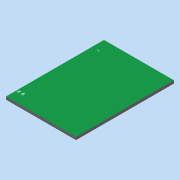
# Autodesk Inventor part: mezzaninePCB
Saved by Autodesk Inventor 2016 (Build 200138000, 138)
## iProperties
Created: 2016-08-31
Part Number: mezzaninePCB
Material: Generic
Document SubType Name: Modeling
Designer: Zara
Density: 1 g/cm^3
Appearance: Default
Author: Zara
Autodesk Inventor part; units mm, degrees
ref_plane "YZ Plane" through (0, 0, 0) normal (1, 0, 0) x (0, 1, 0)
ref_plane "XZ Plane" through (0, 0, 0) normal (0, 1, 0) x (-1, 0, 0)
ref_plane "XY Plane" through (0, 0, 0) normal (0, 0, 1) x (1, 0, 0)
sketch "Sketch1" plane through (0, 0, 0) normal (0, 1, 0) x (-1, 0, 0)
  line L0 (-25, 35) -> (25, 35)
  line L1 (25, 35) -> (25, -35)
  line L2 (25, -35) -> (-25, -35)
  line L3 (-25, -35) -> (-25, 35)
  line L4 (-25, 35) -> (25, -35) construction
  line L5 (25, 35) -> (-25, -35) construction
  point P0 (0, 0)
  dimension "d0" = 70
  dimension "d1" = 50
  constraints: 12 end point, 2 midpoint, 2 parallel, 1 horizontal, 1 perpendicular
  measures "d0" distance of L0.end L1.end
  measures "d1" distance of L1.end L2.end
extrude "Extrusion1" add sketch "Sketch1" along normal blind 2
sketch "Sketch2" plane through (0, 2, 0) normal (0, 1, 0) x (1, 0, 0)
  line L0 (-19.9573, 27.2181) -> (-19.9573, 24.5917) construction
  line L1 (-19.9573, 24.5917) -> (-23.5311, 24.5917) construction
  line L2 (-23.5311, 24.5917) -> (-23.5311, 27.2181) construction
  line L3 (-23.5311, 27.2181) -> (-19.9573, 27.2181) construction
  line L4 (-23.2113, -25.6951) -> (-23.2113, -28.3215) construction
  line L5 (-23.2113, -28.3215) -> (-19.3854, -28.3215) construction
  line L6 (-19.3854, -28.3215) -> (-19.3854, -25.6951) construction
  line L7 (-19.3854, -25.6951) -> (-23.2113, -25.6951) construction
  line L8 (-19.9654, -25.6528) -> (-19.9654, -28.2792) construction
  line L9 (-19.9654, -28.2792) -> (-23.5391, -28.2792) construction
  line L10 (-23.5391, -28.2792) -> (-23.5391, -25.6528) construction
  line L11 (-23.5391, -25.6528) -> (-19.9654, -25.6528) construction
  line L12 (-21.489, 26.1837) -> (-21.489, 27.1087)
  line L13 (-21.489, 27.1087) -> (-21.2762, 27.1087)
  spline S0 degree 2 poles (-21.2762, 27.1087) (-21.1826, 27.0091) (-21.0088, 26.8316) (-20.9152, 26.7465) knots 0 0 0 1 2 2 2
  spline S1 degree 2 poles (-20.9152, 26.7465) (-20.7268, 26.5751) (-20.5007, 26.4499) (-20.3804, 26.4499) knots 0 0 0 1 2 2 2
  spline S2 degree 2 poles (-20.3804, 26.4499) (-20.3172, 26.4499) (-20.2223, 26.4888) (-20.1919, 26.5241) knots 0 0 0 1 2 2 2
  spline S3 degree 2 poles (-20.1919, 26.5241) (-20.1616, 26.5593) (-20.1312, 26.6517) (-20.1312, 26.7076) knots 0 0 0 1 2 2 2
  spline S4 degree 2 poles (-20.1312, 26.7076) (-20.1312, 26.7611) (-20.1579, 26.8705) (-20.1786, 26.9203) knots 0 0 0 1 2 2 2
  spline S5 degree 2 poles (-20.1786, 26.9203) (-20.1956, 26.9629) (-20.2442, 27.0419) (-20.2612, 27.0662) knots 0 0 0 1 2 2 2
  line L14 (-20.2612, 27.0662) -> (-20.2612, 27.0771)
  line L15 (-20.2612, 27.0771) -> (-20.0473, 27.0771)
  spline S6 degree 2 poles (-20.0473, 27.0771) (-20.0169, 27.0151) (-19.9573, 26.7927) (-19.9573, 26.693) knots 0 0 0 1 2 2 2
  spline S7 degree 2 poles (-19.9573, 26.693) (-19.9573, 26.4827) (-20.1798, 26.2457) (-20.3694, 26.2457) knots 0 0 0 1 2 2 2
  spline S8 degree 2 poles (-20.3694, 26.2457) (-20.4582, 26.2457) (-20.6065, 26.287) (-20.6697, 26.3235) knots 0 0 0 1 2 2 2
  spline S9 degree 2 poles (-20.6697, 26.3235) (-20.7353, 26.36) (-20.8642, 26.4657) (-20.9261, 26.5241) knots 0 0 0 1 2 2 2
  spline S10 degree 2 poles (-20.9261, 26.5241) (-21.0295, 26.6189) (-21.2507, 26.851) (-21.3151, 26.9203) knots 0 0 0 1 2 2 2
  line L16 (-21.3151, 26.9203) -> (-21.3151, 26.1837)
  line L17 (-21.3151, 26.1837) -> (-21.489, 26.1837)
  line L18 (-20.9804, -26.7273) -> (-20.9804, -26.5486)
  line L19 (-20.9804, -26.5486) -> (-21.4958, -26.5486)
  line L20 (-21.4958, -26.5486) -> (-21.4958, -26.3554)
  line L21 (-21.4958, -26.3554) -> (-20.9804, -26.3554)
  line L22 (-20.9804, -26.3554) -> (-20.9804, -25.6929)
  line L23 (-20.9804, -25.6929) -> (-20.7689, -25.6929)
  line L24 (-20.7689, -25.6929) -> (-19.9958, -26.3639)
  line L25 (-19.9958, -26.3639) -> (-19.9958, -26.5486)
  line L26 (-19.9958, -26.5486) -> (-20.8187, -26.5486)
  line L27 (-20.8187, -26.5486) -> (-20.8187, -26.7273)
  line L28 (-20.8187, -26.7273) -> (-20.9804, -26.7273)
  line L29 (-20.8187, -26.3554) -> (-20.2328, -26.3554)
  line L30 (-20.2328, -26.3554) -> (-20.8187, -25.8509)
  line L31 (-20.8187, -25.8509) -> (-20.8187, -26.3554)
  spline S11 degree 2 poles (-20.7458, -27.8213) (-21.1493, -27.8213) (-21.5274, -27.5867) (-21.5274, -27.3424) knots 0 0 0 1 2 2 2
  spline S12 degree 2 poles (-21.5274, -27.3424) (-21.5274, -27.0944) (-21.142, -26.8622) (-20.747, -26.8622) knots 0 0 0 1 2 2 2
  spline S13 degree 2 poles (-20.747, -26.8622) (-20.341, -26.8622) (-19.9654, -27.0969) (-19.9654, -27.3424) knots 0 0 0 1 2 2 2
  spline S14 degree 2 poles (-19.9654, -27.3424) (-19.9654, -27.5892) (-20.3544, -27.8213) (-20.7458, -27.8213) knots 0 0 0 1 2 2 2
  spline S15 degree 2 poles (-21.2028, -27.5636) (-21.1287, -27.5928) (-20.9002, -27.6171) (-20.7458, -27.6171) knots 0 0 0 1 2 2 2
  spline S16 degree 2 poles (-20.7458, -27.6171) (-20.5914, -27.6171) (-20.3641, -27.5928) (-20.2875, -27.5624) knots 0 0 0 1 2 2 2
  spline S17 degree 2 poles (-20.2875, -27.5624) (-20.2109, -27.532) (-20.1319, -27.4263) (-20.1319, -27.3424) knots 0 0 0 1 2 2 2
  spline S18 degree 2 poles (-20.1319, -27.3424) (-20.1319, -27.2585) (-20.2109, -27.1503) (-20.2899, -27.1187) knots 0 0 0 1 2 2 2
  spline S19 degree 2 poles (-20.2899, -27.1187) (-20.3665, -27.0883) (-20.5999, -27.0665) (-20.747, -27.0665) knots 0 0 0 1 2 2 2
  spline S20 degree 2 poles (-20.747, -27.0665) (-20.905, -27.0665) (-21.1165, -27.0859) (-21.1992, -27.1175) knots 0 0 0 1 2 2 2
  spline S21 degree 2 poles (-21.1992, -27.1175) (-21.277, -27.1467) (-21.3608, -27.2549) (-21.3608, -27.3424) knots 0 0 0 1 2 2 2
  spline S22 degree 2 poles (-21.3608, -27.3424) (-21.3608, -27.4251) (-21.2818, -27.5332) (-21.2028, -27.5636) knots 0 0 0 1 2 2 2
  spline S23 degree 2 poles (-23.3852, -26.2093) (-23.3852, -26.1546) (-23.4119, -26.0464) (-23.4326, -25.9941) knots 0 0 0 1 2 2 2
  spline S24 degree 2 poles (-23.4326, -25.9941) (-23.4532, -25.9455) (-23.497, -25.8738) (-23.5165, -25.8458) knots 0 0 0 1 2 2 2
  line L32 (-23.5165, -25.8458) -> (-23.5165, -25.8337)
  line L33 (-23.5165, -25.8337) -> (-23.3037, -25.8337)
  spline S25 degree 2 poles (-23.3037, -25.8337) (-23.2685, -25.8993) (-23.2113, -26.1242) (-23.2113, -26.2251) knots 0 0 0 1 2 2 2
  spline S26 degree 2 poles (-23.2113, -26.2251) (-23.2113, -26.3272) (-23.2527, -26.4791) (-23.2964, -26.5411) knots 0 0 0 1 2 2 2
  spline S27 degree 2 poles (-23.2964, -26.5411) (-23.3438, -26.6067) (-23.4812, -26.6748) (-23.5736, -26.6748) knots 0 0 0 1 2 2 2
  spline S28 degree 2 poles (-23.5736, -26.6748) (-23.6976, -26.6748) (-23.8848, -26.5119) (-23.9091, -26.3977) knots 0 0 0 1 2 2 2
  line L34 (-23.9091, -26.3977) -> (-23.9237, -26.3977)
  spline S29 degree 2 poles (-23.9237, -26.3977) (-23.9334, -26.4451) (-23.9771, -26.5533) (-24.0209, -26.5995) knots 0 0 0 1 2 2 2
  spline S30 degree 2 poles (-24.0209, -26.5995) (-24.0635, -26.6456) (-24.1996, -26.704) (-24.2981, -26.704) knots 0 0 0 1 2 2 2
  spline S31 degree 2 poles (-24.2981, -26.704) (-24.3989, -26.704) (-24.5703, -26.6347) (-24.636, -26.5715) knots 0 0 0 1 2 2 2
  spline S32 degree 2 poles (-24.636, -26.5715) (-24.7041, -26.5059) (-24.7746, -26.3199) (-24.7746, -26.202) knots 0 0 0 1 2 2 2
  spline S33 degree 2 poles (-24.7746, -26.202) (-24.7746, -26.0889) (-24.7199, -25.8677) (-24.6822, -25.7923) knots 0 0 0 1 2 2 2
  line L35 (-24.6822, -25.7923) -> (-24.4694, -25.7923)
  line L36 (-24.4694, -25.7923) -> (-24.4694, -25.8069)
  spline S34 degree 2 poles (-24.4694, -25.8069) (-24.5156, -25.8701) (-24.6007, -26.0841) (-24.6007, -26.1898) knots 0 0 0 1 2 2 2
  spline S35 degree 2 poles (-24.6007, -26.1898) (-24.6007, -26.2518) (-24.5618, -26.3758) (-24.5169, -26.4171) knots 0 0 0 1 2 2 2
  spline S36 degree 2 poles (-24.5169, -26.4171) (-24.4719, -26.4572) (-24.3649, -26.4998) (-24.2835, -26.4998) knots 0 0 0 1 2 2 2
  spline S37 degree 2 poles (-24.2835, -26.4998) (-24.202, -26.4998) (-24.0963, -26.4524) (-24.0659, -26.4098) knots 0 0 0 1 2 2 2
  spline S38 degree 2 poles (-24.0659, -26.4098) (-24.0355, -26.3673) (-24.0124, -26.2518) (-24.0124, -26.1837) knots 0 0 0 1 2 2 2
  line L37 (-24.0124, -26.1837) -> (-24.0124, -26.0986)
  line L38 (-24.0124, -26.0986) -> (-23.8459, -26.0986)
  line L39 (-23.8459, -26.0986) -> (-23.8459, -26.1655)
  spline S39 degree 2 poles (-23.8459, -26.1655) (-23.8459, -26.3004) (-23.717, -26.4706) (-23.5942, -26.4706) knots 0 0 0 1 2 2 2
  spline S40 degree 2 poles (-23.5942, -26.4706) (-23.5371, -26.4706) (-23.4557, -26.4268) (-23.4314, -26.3916) knots 0 0 0 1 2 2 2
  spline S41 degree 2 poles (-23.4314, -26.3916) (-23.4058, -26.3539) (-23.3852, -26.2615) (-23.3852, -26.2093) knots 0 0 0 1 2 2 2
  spline S42 degree 2 poles (-23.7304, -26.8888) (-23.6149, -26.8888) (-23.4229, -26.9641) (-23.3536, -27.0298) knots 0 0 0 1 2 2 2
  spline S43 degree 2 poles (-23.3536, -27.0298) (-23.2867, -27.0918) (-23.2126, -27.2729) (-23.2126, -27.3653) knots 0 0 0 1 2 2 2
  spline S44 degree 2 poles (-23.2126, -27.3653) (-23.2126, -27.4686) (-23.2818, -27.6363) (-23.3475, -27.6983) knots 0 0 0 1 2 2 2
  spline S45 degree 2 poles (-23.3475, -27.6983) (-23.4301, -27.7761) (-23.6976, -27.8612) (-23.903, -27.8612) knots 0 0 0 1 2 2 2
  spline S46 degree 2 poles (-23.903, -27.8612) (-24.089, -27.8612) (-24.422, -27.7773) (-24.5327, -27.6959) knots 0 0 0 1 2 2 2
  spline S47 degree 2 poles (-24.5327, -27.6959) (-24.6494, -27.6096) (-24.7721, -27.3665) (-24.7721, -27.189) knots 0 0 0 1 2 2 2
  spline S48 degree 2 poles (-24.7721, -27.189) (-24.7721, -27.1489) (-24.7636, -27.0577) (-24.7515, -27.0188) knots 0 0 0 1 2 2 2
  line L40 (-24.7515, -27.0188) -> (-24.5582, -27.0188)
  line L41 (-24.5582, -27.0188) -> (-24.5582, -27.0285)
  spline S49 degree 2 poles (-24.5582, -27.0285) (-24.5728, -27.0541) (-24.5983, -27.161) (-24.5983, -27.2157) knots 0 0 0 1 2 2 2
  spline S50 degree 2 poles (-24.5983, -27.2157) (-24.5983, -27.4127) (-24.3382, -27.6375) (-24.0975, -27.6533) knots 0 0 0 1 2 2 2
  spline S51 degree 2 poles (-24.0975, -27.6533) (-24.1522, -27.5731) (-24.202, -27.4272) (-24.202, -27.3409) knots 0 0 0 1 2 2 2
  spline S52 degree 2 poles (-24.202, -27.3409) (-24.202, -27.2583) (-24.1656, -27.1209) (-24.1133, -27.0516) knots 0 0 0 1 2 2 2
  spline S53 degree 2 poles (-24.1133, -27.0516) (-24.0513, -26.9714) (-23.8629, -26.8888) (-23.7304, -26.8888) knots 0 0 0 1 2 2 2
  spline S54 degree 2 poles (-23.858, -27.6582) (-23.7061, -27.6582) (-23.514, -27.6023) (-23.4618, -27.5525) knots 0 0 0 1 2 2 2
  spline S55 degree 2 poles (-23.4618, -27.5525) (-23.4131, -27.5087) (-23.3767, -27.4175) (-23.3767, -27.364) knots 0 0 0 1 2 2 2
  spline S56 degree 2 poles (-23.3767, -27.364) (-23.3767, -27.2401) (-23.5541, -27.093) (-23.7219, -27.093) knots 0 0 0 1 2 2 2
  spline S57 degree 2 poles (-23.7219, -27.093) (-23.8167, -27.093) (-23.9395, -27.1416) (-23.9832, -27.1951) knots 0 0 0 1 2 2 2
  spline S58 degree 2 poles (-23.9832, -27.1951) (-24.0148, -27.234) (-24.0355, -27.33) (-24.0355, -27.3859) knots 0 0 0 1 2 2 2
  spline S59 degree 2 poles (-24.0355, -27.3859) (-24.0355, -27.4503) (-23.9905, -27.5986) (-23.9528, -27.6546) knots 0 0 0 1 2 2 2
  spline S60 degree 2 poles (-23.9528, -27.6546) (-23.9382, -27.6558) (-23.8884, -27.6582) (-23.858, -27.6582) knots 0 0 0 1 2 2 2
  point P0 (0, 0)
  constraints: 6 other
emboss "Emboss1" sketch "Sketch2" operation add depth 1 direction (0, -1, 0)
body "Solid1"
